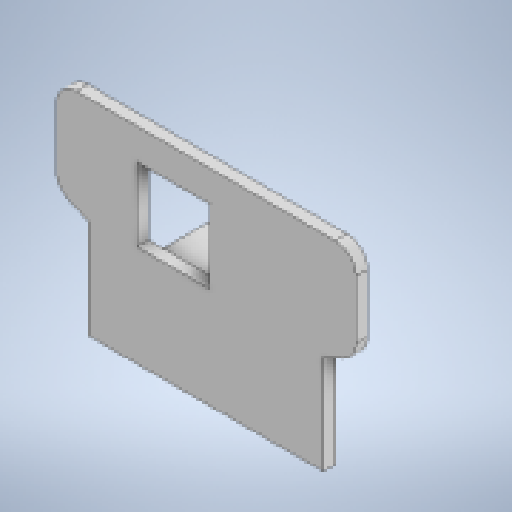
# Autodesk Inventor part: top_closure
Saved by Autodesk Inventor 2023.3 (Build 273359000, 359)
## iProperties
Created: 2023-07-28
Part Number: top_closure
Material: Generic
Document SubType Name: Modeling
Designer: mmelin
Density: 1 g/cm^3
Appearance: Default
Author: mmelin
Autodesk Inventor part; units mm, degrees
ref_plane "YZ Plane" through (0, 0, 0) normal (1, 0, 0) x (0, 1, 0)
ref_plane "XZ Plane" through (0, 0, 0) normal (0, 1, 0) x (-1, 0, 0)
ref_plane "XY Plane" through (0, 0, 0) normal (0, 0, 1) x (1, 0, 0)
sketch "Sketch1" plane through (0, 0, 0) normal (0, 0, 1) x (1, 0, 0)
  arc A0 (-4.8, 0.55) -> (-5.6, -0.25) centre (-4.8, -0.25) ccw projected
  line L0 (-5.6, -2.6349) -> (-5.6, -0.25) projected
  arc A1 (-5.6, -2.6349) -> (-5.3449, -3.2206) centre (-4.8, -2.6349) ccw projected
  arc A2 (-5.1931, -3.4997) -> (-5.3449, -3.2206) centre (-5.6855, -3.5867) ccw projected
  line L1 (-5.1931, -3.4997) -> (-4.6759, -3.7348) projected
  line L2 (-4.5, -7.45) -> (-4.5, -4.0079) projected
  line L3 (4.5, -7.45) -> (-4.5, -7.45) projected
  line L4 (4.5, -3.9927) -> (4.5, -7.45) projected
  line L5 (4.7986, -3.679) -> (5.1931, -3.4997) projected
  arc A3 (5.3449, -3.2206) -> (5.1931, -3.4997) centre (5.6855, -3.5867) ccw projected
  arc A4 (5.3449, -3.2206) -> (5.6, -2.6349) centre (4.8, -2.6349) ccw projected
  line L6 (5.6, -2.6349) -> (5.6, -0.25) projected
  arc A5 (5.6, -0.25) -> (4.8, 0.55) centre (4.8, -0.25) ccw projected
  line L7 (-4.8, 0.55) -> (4.8, 0.55) projected
  line L8 (-4.1, -3.65) -> (-4.731, -3.3632) projected
  arc A6 (-5.2, -2.6349) -> (-4.731, -3.3632) centre (-4.4, -2.6349) ccw projected
  line L9 (-5.2, -2.6349) -> (-5.2, -0.65) projected
  arc A7 (-4.4, 0.15) -> (-5.2, -0.65) centre (-4.4, -0.65) ccw projected
  line L10 (-4.4, 0.15) -> (4.4, 0.15) projected
  arc A8 (5.2, -0.65) -> (4.4, 0.15) centre (4.4, -0.65) ccw projected
  line L11 (5.2, -2.6349) -> (5.2, -0.65) projected
  arc A9 (4.731, -3.3632) -> (5.2, -2.6349) centre (4.4, -2.6349) ccw projected
  line L12 (4.731, -3.3632) -> (4.1, -3.65) projected
  line L13 (4.1, -7.05) -> (4.1, -3.65) projected
  line L14 (-4.1, -7.05) -> (4.1, -7.05) projected
  line L15 (-4.1, -3.65) -> (-4.1, -7.05) projected
  line L16 (-4, -6.95) -> (4, -6.95)
  line L17 (4, -6.95) -> (4, -3.5856)
  arc A10 (5.1, -0.65) -> (4.4, 0.05) centre (4.4, -0.65) ccw
  line L18 (5.1, -2.6349) -> (5.1, -0.65)
  line L19 (4.4, 0.05) -> (-4.4, 0.05)
  line L20 (4, -3.5856) -> (4.6897, -3.2721)
  arc A11 (4.6897, -3.2721) -> (5.1, -2.6349) centre (4.4, -2.6349) ccw
  line L21 (-4, -6.95) -> (-4, -3.5856)
  line L22 (-4, -3.5856) -> (-4.6897, -3.2721)
  line L23 (-5.1, -2.6349) -> (-5.1, -0.65)
  arc A12 (-5.1, -2.6349) -> (-4.6897, -3.2721) centre (-4.4, -2.6349) ccw
  arc A13 (-4.4, 0.05) -> (-5.1, -0.65) centre (-4.4, -0.65) ccw
  arc A14 (4.7372, -3.6993) -> (4.7986, -3.679) centre (4.6744, -3.4059) ccw projected
  arc A15 (4.7372, -3.6993) -> (4.5, -3.9927) centre (4.8, -3.9927) ccw projected
  arc A16 (-4.5, -4.0079) -> (-4.6759, -3.7348) centre (-4.8, -4.0079) ccw projected
  point P0 (0, 0)
  dimension "d1" = 0.1
  dimension "d2" = 0.1
  dimension "d3" = 0.1
  dimension "d4" = 0.1
  dimension "d5" = 0.1
  dimension "d7" = 0.1
  dimension "d8" = 0.1
  dimension "d9" = 0.1
  dimension "d10" = 0.1
  dimension "d11" = 0.1
  dimension "d13" = 0.1
  dimension "d15" = 0.1
  constraints: 16 end point, 8 point on circle, 6 parallel, 4 centre point, 4 coincident, 2 horizontal, 2 vertical
  measures "d1" distance between parallel lines of L14 L16
  measures "d2" distance between parallel lines of L13 L17
  measures "d3" distance between parallel lines of L12 L20
  measures "d4" distance between parallel lines of L11 L18
  measures "d5" distance between parallel lines of L10 L19
  measures "d7" radial gap between concentric circles of A8 A10
  measures "d8" radial gap between concentric circles of A9 A11
  measures "d9" distance between parallel lines of L15 L21
  measures "d10" distance between parallel lines of L8 L22
  measures "d11" distance between parallel lines of L9 L23
  measures "d13" radial gap between concentric circles of A6 A12
  measures "d15" radial gap between concentric circles of A7 A13
extrude "Extrusion1" add sketch "Sketch1" along normal blind 0.4 contours L21 L22 A12 L23 A13 L19 A10 L18 A11 L20 L17 L16
sketch "Sketch2" plane through (0, 0, 0.4) normal (0, 0, 1) x (1, 0, 0)
  line L0 (0.15, -3.5039) -> (-2.35, -3.5039)
  line L1 (-2.35, -3.5039) -> (-2.35, -1.0039)
  line L2 (-2.35, -1.0039) -> (0.15, -1.0039)
  line L3 (0.15, -1.0039) -> (0.15, -3.5039)
  line L4 (4.4, 0.05) -> (-4.4, 0.05) projected
  line L5 (-5.1, -0.65) -> (-5.1, -2.6349) projected
  line L6 (5.1, -2.6349) -> (5.1, -0.65) projected
  point P0 (0, 0)
  dimension "d18" = 1.0539
  dimension "d19" = 2.75
  dimension "d21" = 2.5
  dimension "d22" = 4.95
  dimension "d23" = 2.5
  constraints: 8 end point, 2 parallel, 1 horizontal, 1 perpendicular
  measures "d18" distance between parallel lines of L4 L2
  measures "d19" distance between parallel lines of L5 L1
  measures "d21" distance of L2.end L0.start
  measures "d22" distance between parallel lines of L6 L3
  measures "d23" distance of L0.start L0.end
extrude "Extrusion2" cut sketch "Sketch2" against normal up to surface (0.4 mm away)
sketch "Sketch3" plane through (0, 0, 0) normal (0, 0, -1) x (-1, 0, 0)
  line L0 (-1.0895, -3.95) -> (2.3023, -3.95)
  line L1 (2.3023, -3.95) -> (2.3023, -4.35)
  line L2 (2.3023, -4.35) -> (-1.0895, -4.35)
  line L3 (-1.0895, -4.35) -> (-1.0895, -3.95)
  line L4 (-4.4, 0.05) -> (4.4, 0.05) projected
  point P0 (0, 0)
  dimension "d28" = 4
  dimension "d29" = 0.4
  constraints: 8 end point, 2 parallel, 1 horizontal, 1 perpendicular
  measures "d28" distance between parallel lines of L0 L4
  measures "d29" distance of L0.end L1.end
extrude "Extrusion3" add sketch "Sketch3" along normal blind 3
equation "\"d2\" = d1"
equation "\"d3\" = d1"
equation "\"d4\" = d2"
equation "\"d5\" = d1"
equation "\"d7\" = d4"
equation "\"d8\" = d2"
equation "\"d9\" = d1"
equation "\"d10\" = d9"
equation "\"d11\" = d10"
body "Solid1"
